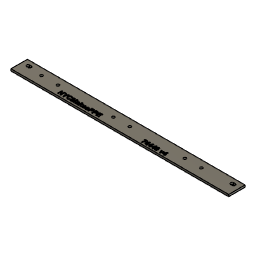
74440 verk v4 (Autodesk Fusion 360 design; units mm, degrees)
Autodesk Fusion 360 part; units mm, degrees
sketch "Sketch1" plane through (0, 0, 0) normal (0, 1, 0) x (1, 0, 0)
  line L0 (0, 0) -> (330.2, 0)
  line L1 (330.2, 0) -> (330.2, 25.4)
  line L2 (330.2, 25.4) -> (0, 25.4)
  line L3 (0, 25.4) -> (0, 0)
  circle A0 centre (9.1, 17.3) radius 2.25
  circle A1 centre (29.8, 14.5) radius 2.05
  circle A2 centre (55.2, 14.5) radius 2.05
  circle A3 centre (140.8, 14.5) radius 2.05
  circle A4 centre (166.2, 14.5) radius 2.05
  circle A5 centre (251.2, 14.5) radius 2.05
  circle A6 centre (276.6, 14.5) radius 2.05
  circle A7 centre (321.1, 17.3) radius 2.25
  circle A8 centre (324.1, 17.3) radius 2.25
  line L4 (321.1, 19.55) -> (324.1, 19.55)
  line L5 (321.1, 15.05) -> (324.1, 15.05)
  circle A9 centre (6.1, 17.3) radius 2.25
  line L6 (6.1, 19.55) -> (9.1, 19.55)
  line L7 (6.1, 15.05) -> (9.1, 15.05)
  dimension "d1" = 330.2
  dimension "d2" = 25.4
  dimension "d3" = 4.5
  dimension "d4" = 8.1
  dimension "d5" = 9.1
  dimension "d6" = 4.1
  dimension "d7" = 10.9
  dimension "d8" = 29.8
  dimension "d9" = 55.2
  dimension "d10" = 140.8
  dimension "d11" = 166.2
  dimension "d13" = 251.2
  dimension "d14" = 276.6
  dimension "d15" = 321.1
  dimension "d27" = 3
  dimension "d28" = 3
  constraint horizontal L0
  constraint vertical L1
  constraint horizontal L2
  constraint vertical L3
  constraint coincident L0.start L3.end
  constraint equal A1 A2
  constraint horizontal A1.centre A2.centre
  constraint equal A2 A3
  constraint horizontal A2.centre A3.centre
  constraint equal A3 A4
  constraint horizontal A3.centre A4.centre
  constraint equal A4 A5
  constraint horizontal A4.centre A5.centre
  constraint equal A5 A6
  constraint horizontal A5.centre A6.centre
  constraint equal A0 A7
  constraint horizontal A0.centre A7.centre
  constraint equal A7 A8
  constraint horizontal A7.centre A8.centre
  constraint horizontal L4
  constraint tangent A8 L4
  constraint coincident A7 L4.start
  constraint coincident A8 L4.end
  constraint horizontal L5
  constraint tangent A7 L5
  constraint coincident A8 L5.end
  constraint coincident A7 L5.start
  constraint equal A0 A9
  constraint horizontal A0.centre A9.centre
  constraint horizontal L6
  constraint coincident A9 L6.start
  constraint tangent A9 L6
  constraint coincident A0 L6.end
  constraint horizontal L7
  constraint coincident A9 L7.start
  constraint tangent A9 L7
  constraint coincident A0 L7.end
  measures "d1" distance of L0.start L0.end
  measures "d2" distance of L0.start L2.end
  measures "d3" diameter of A0
  measures "d4" distance of L2 A0.centre
  measures "d5" distance of L3 A0.centre
  measures "d6" diameter of A1
  measures "d7" distance of L2 A1.centre
  measures "d8" distance of L3 A1.centre
  measures "d9" distance of L3 A2.centre
  measures "d10" distance of L3 A3.centre
  measures "d11" distance of L3 A4.centre
  measures "d13" distance of L3 A5.centre
  measures "d14" distance of L3 A6.centre
  measures "d15" distance of L3 A7.centre
  measures "d27" distance of A7.centre A8.centre
  measures "d28" distance of A0.centre A9.centre
extrude "Extrude1" add sketch "Sketch1" along normal blind 3
sketch "Sketch2" plane through (0, 3, 0) normal (0, 1, 0) x (-1, 0, 0)
  circle A0 centre (-276.6, -14.5) radius 2.05
  circle A1 centre (-251.2, -14.5) radius 2.05
  circle A2 centre (-166.2, -14.5) radius 2.05
  circle A3 centre (-140.8, -14.5) radius 2.05
  circle A4 centre (-55.2, -14.5) radius 2.05
  circle A5 centre (-29.8, -14.5) radius 2.05
  line L0 (0, -25.4) -> (0, 0)
  line L1 (0, 0) -> (-330.2, 0)
  line L2 (-330.2, 0) -> (-330.2, -25.4)
  line L3 (-330.2, -25.4) -> (0, -25.4)
  line L4 (-65.6223, -3.3986) -> (-129.0354, -3.3986) construction
  line L5 (-129.0354, -3.3986) -> (-129.0354, -12.3986) construction
  line L6 (-129.0354, -12.3986) -> (-65.6223, -12.3986) construction
  line L7 (-65.6223, -12.3986) -> (-65.6223, -3.3986) construction
  line L8 (-194.7512, -2.5925) -> (-231.7004, -2.5925) construction
  line L9 (-231.7004, -2.5925) -> (-231.7004, -11.5925) construction
  line L10 (-231.7004, -11.5925) -> (-194.7512, -11.5925) construction
  line L11 (-194.7512, -11.5925) -> (-194.7512, -2.5925) construction
  arc A6 (-6.1, -19.55) -> (-6.1, -15.05) centre (-6.1, -17.3) ccw
  line L12 (-6.1, -19.55) -> (-9.1, -19.55)
  arc A7 (-9.1, -15.05) -> (-9.1, -19.55) centre (-9.1, -17.3) ccw
  line L13 (-9.1, -15.05) -> (-6.1, -15.05)
  arc A8 (-321.1, -19.55) -> (-321.1, -15.05) centre (-321.1, -17.3) ccw
  line L14 (-321.1, -19.55) -> (-324.1, -19.55)
  arc A9 (-324.1, -15.05) -> (-324.1, -19.55) centre (-324.1, -17.3) ccw
  line L15 (-324.1, -15.05) -> (-321.1, -15.05)
  text T0 "NYCMakesPPE" font "Arial" height 9 bold align ink ink in box 0 x 0 at (-65.6323, -3.4186) x (-1, 0) y (0, -1) spacing 1 height is em
  text T1 "74440 v4" font "Arial" height 9 bold align ink ink in box 0 x 0 at (-194.7612, -2.6125) x (-1, 0) y (0, -1) spacing 1 height is em
  constraint perpendicular L4 L5
  constraint parallel L4 L6
  constraint parallel L5 L7
  constraint perpendicular L8 L9
  constraint parallel L8 L10
  constraint parallel L9 L11
extrude "Extrude3" cut sketch "Sketch2" against normal blind 1 text T1 T0
extrude "Extrude4" add 1 faces at (0, 1, -16.9333) along direction (-1, 0, 0) blind 3
extrude "Extrude5" add 1 faces at (330.2, 1, -8.4667) along direction (1, 0, 0) blind 3
equation "d10 = 137.8 mm + 3 mm"
equation "d11 = 163.2 mm + 3 mm"
equation "d13 = 245.7 mm + 5.5 mm"
equation "d14 = 271.1 mm + 5.5 mm"
